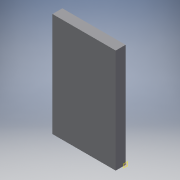
# Autodesk Inventor part: seat
Saved by Autodesk Inventor 2016 SP1 (Build 200210100, 210)
## iProperties
Created: 2016-06-25
Part Number: seat
Material: Generic
Document SubType Name: Modeling
Designer: asvsf
Density: 1 g/cm^3
Appearance: Default
Author: asvsf
Autodesk Inventor part; units mm, degrees
ref_plane "YZ Plane" through (0, 0, 0) normal (1, 0, 0) x (0, 1, 0)
ref_plane "XZ Plane" through (0, 0, 0) normal (0, 1, 0) x (-1, 0, 0)
ref_plane "XY Plane" through (0, 0, 0) normal (0, 0, 1) x (1, 0, 0)
sketch "Sketch1" plane through (0, 0, 0) normal (0, 1, 0) x (-1, 0, 0)
  line L0 (29.7115, -23.0055) -> (-325.8885, -23.0055)
  line L1 (-325.8885, -23.0055) -> (-325.8885, 357.9945)
  line L2 (-325.8885, 357.9945) -> (29.7115, 357.9945)
  line L3 (29.7115, 357.9945) -> (29.7115, -23.0055)
  line L4 (29.7115, 32.7) -> (-325.8885, 32.7)
  point P0 (0, 0)
  dimension "d0" = 355.6
  dimension "d1" = 381
  constraints: 10 end point, 4 perpendicular, 2 point on line, 1 horizontal
  measures "d0" distance of L0.start L0.end
  measures "d1" distance of L0.end L1.end
ref_plane "Work Plane2" through (325.8885, 0, -23.0055) normal (1, 0, 0) x (0, 1, 0)
extrude "Extrusion1" add sketch "Sketch1" along normal blind 584.2 contours L0 L1 L4 L3
body "Solid1"
